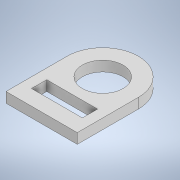
# Autodesk Inventor part: Exercise_1
Saved by Autodesk Inventor 2020 (Build 240168000, 168)
## iProperties
Created: 2022-11-07
Part Number: Exercise_1
Material: Generic
Document SubType Name: Modeling
Designer: Matthew Ng
Density: 1 g/cm^3
Appearance: Default
Author: Matthew Ng
Autodesk Inventor part; units mm, degrees
ref_plane "YZ Plane" through (0, 0, 0) normal (1, 0, 0) x (0, 1, 0)
ref_plane "XZ Plane" through (0, 0, 0) normal (0, 1, 0) x (-1, 0, 0)
ref_plane "XY Plane" through (0, 0, 0) normal (0, 0, 1) x (1, 0, 0)
sketch "Sketch1" plane through (0, 0, 0) normal (0, 1, 0) x (-1, 0, 0)
  line L0 (0, 0) -> (-70, 0)
  line L1 (-70, 0) -> (-70, -60)
  line L2 (0, -60) -> (0, 0)
  arc A0 (-70, -60) -> (0, -60) centre (-35, -60) ccw
  circle A1 centre (-35, -60) radius 20
  line L3 (-10, -15) -> (-60, -15)
  line L4 (-60, -15) -> (-60, -30)
  line L5 (-60, -30) -> (-10, -30)
  line L6 (-10, -30) -> (-10, -15)
  dimension "d0" = 70
  dimension "d1" = 60
  dimension "d4" = 40
  dimension "d6" = 50
  dimension "d7" = 15
  dimension "d8" = 15
  dimension "d9" = 10
  constraints: 14 end point, 3 parallel, 2 centre point, 2 horizontal, 2 perpendicular, 2 point on circle, 1 coincident
  measures "d0" distance of L2.start L1.end
  measures "d1" distance of L1.end L0.end
  measures "d4" diameter of A1
  measures "d6" distance of L5.end L4.end
  measures "d7" distance of L4.end L3.end
  measures "d8" distance between parallel lines of L0 L3
  measures "d9" distance between parallel lines of L2 L6
extrude "Extrusion1" add sketch "Sketch1" along normal blind 10
body "Solid1"
